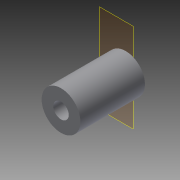
# Autodesk Inventor part: wheel spacers
Saved by Autodesk Inventor 2015 (Build 190159000, 159)
## iProperties
Created: 2014-10-11
Part Number: wheel spacers
Material: Generic
Document SubType Name: Modeling
Designer: jesse
Density: 1 g/cm^3
Appearance: Default
Author: jesse
Autodesk Inventor part; units mm, degrees
ref_plane "YZ Plane" through (0, 0, 0) normal (1, 0, 0) x (0, 1, 0)
ref_plane "XZ Plane" through (0, 0, 0) normal (0, 1, 0) x (-1, 0, 0)
ref_plane "XY Plane" through (0, 0, 0) normal (0, 0, 1) x (1, 0, 0)
ref_plane "Work Plane1" through (0, 0, 0) normal (0, 0, 1) x (1, 0, 0)
sketch "Sketch1" plane through (0, 0, 0) normal (0, 0, 1) x (1, 0, 0)
  arc A0 (4.2768, 1.4222) -> (4.2768, -1.4222) centre (2.4226, 0) ccw construction
  circle A1 centre (2.4226, 0) radius 2.3795
  circle A2 centre (2.4226, 0) radius 5.9756
  point P0 (0, 0)
  constraints: 2 centre point, 2 coincident
extrude "Extrusion1" add sketch "Sketch1" along normal blind 33.5928
body "Solid1"
